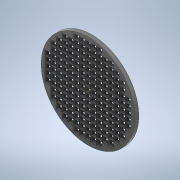
# Autodesk Inventor part: FRAME
Saved by Autodesk Inventor 2022 (Build 260153000, 153)
## iProperties
Created: 2022-02-07
Part Number: FRAME
Material: Copper
Document SubType Name: Modeling
Designer: joshw
Density: 8.94 g/cm^3
Appearance: Diamond plate - Dark Gray
Author: joshw
Autodesk Inventor part; units mm, degrees
ref_plane "YZ Plane" through (0, 0, 0) normal (1, 0, 0) x (0, 1, 0)
ref_plane "XZ Plane" through (0, 0, 0) normal (0, 1, 0) x (-1, 0, 0)
ref_plane "XY Plane" through (0, 0, 0) normal (0, 0, 1) x (1, 0, 0)
sketch "Sketch5" plane through (0, 0, 0) normal (0, 0, 1) x (1, 0, 0)
  line L0 (115, 115) -> (115, -115) construction
  line L1 (115, -115) -> (-115, -115)
  line L2 (-115, -115) -> (-115, 115)
  line L3 (97.5, -97.5) -> (97.5, -111.5)
  line L4 (97.5, -111.5) -> (111.5, -111.5)
  line L5 (111.5, -111.5) -> (111.5, -97.5)
  line L6 (111.5, -97.5) -> (97.5, -97.5)
  line L7 (115, 115) -> (-115, 115)
  line L8 (97.5, -82.5) -> (97.5, -96.5)
  line L9 (97.5, -96.5) -> (111.5, -96.5)
  line L10 (111.5, -96.5) -> (111.5, -82.5)
  line L11 (111.5, -82.5) -> (97.5, -82.5)
  line L12 (97.5, -67.5) -> (97.5, -81.5)
  line L13 (97.5, -81.5) -> (111.5, -81.5)
  line L14 (111.5, -81.5) -> (111.5, -67.5)
  line L15 (111.5, -67.5) -> (97.5, -67.5)
  line L16 (97.5, -52.5) -> (97.5, -66.5)
  line L17 (97.5, -66.5) -> (111.5, -66.5)
  line L18 (111.5, -66.5) -> (111.5, -52.5)
  line L19 (111.5, -52.5) -> (97.5, -52.5)
  line L20 (97.5, -37.5) -> (97.5, -51.5)
  line L21 (97.5, -51.5) -> (111.5, -51.5)
  line L22 (111.5, -51.5) -> (111.5, -37.5)
  line L23 (111.5, -37.5) -> (97.5, -37.5)
  line L24 (97.5, -22.5) -> (97.5, -36.5)
  line L25 (97.5, -36.5) -> (111.5, -36.5)
  line L26 (111.5, -36.5) -> (111.5, -22.5)
  line L27 (111.5, -22.5) -> (97.5, -22.5)
  line L28 (97.5, -7.5) -> (97.5, -21.5)
  line L29 (97.5, -21.5) -> (111.5, -21.5)
  line L30 (111.5, -21.5) -> (111.5, -7.5)
  line L31 (111.5, -7.5) -> (97.5, -7.5)
  line L32 (97.5, 7.5) -> (97.5, -6.5)
  line L33 (97.5, -6.5) -> (111.5, -6.5)
  line L34 (111.5, -6.5) -> (111.5, 7.5)
  line L35 (111.5, 7.5) -> (97.5, 7.5)
  line L36 (97.5, 22.5) -> (97.5, 8.5)
  line L37 (97.5, 8.5) -> (111.5, 8.5)
  line L38 (111.5, 8.5) -> (111.5, 22.5)
  line L39 (111.5, 22.5) -> (97.5, 22.5)
  line L40 (97.5, 37.5) -> (97.5, 23.5)
  line L41 (97.5, 23.5) -> (111.5, 23.5)
  line L42 (111.5, 23.5) -> (111.5, 37.5)
  line L43 (111.5, 37.5) -> (97.5, 37.5)
  line L44 (97.5, 52.5) -> (97.5, 38.5)
  line L45 (97.5, 38.5) -> (111.5, 38.5)
  line L46 (111.5, 38.5) -> (111.5, 52.5)
  line L47 (111.5, 52.5) -> (97.5, 52.5)
  line L48 (97.5, 67.5) -> (97.5, 53.5)
  line L49 (97.5, 53.5) -> (111.5, 53.5)
  line L50 (111.5, 53.5) -> (111.5, 67.5)
  line L51 (111.5, 67.5) -> (97.5, 67.5)
  line L52 (97.5, 82.5) -> (97.5, 68.5)
  line L53 (97.5, 68.5) -> (111.5, 68.5)
  line L54 (111.5, 68.5) -> (111.5, 82.5)
  line L55 (111.5, 82.5) -> (97.5, 82.5)
  line L56 (97.5, 97.5) -> (97.5, 83.5)
  line L57 (97.5, 83.5) -> (111.5, 83.5)
  line L58 (111.5, 83.5) -> (111.5, 97.5)
  line L59 (111.5, 97.5) -> (97.5, 97.5)
  line L60 (97.5, 112.5) -> (97.5, 98.5)
  line L61 (97.5, 98.5) -> (111.5, 98.5)
  line L62 (111.5, 98.5) -> (111.5, 112.5)
  line L63 (111.5, 112.5) -> (97.5, 112.5)
  line L64 (82.5, -97.5) -> (82.5, -111.5)
  line L65 (82.5, -111.5) -> (96.5, -111.5)
  line L66 (96.5, -111.5) -> (96.5, -97.5)
  line L67 (96.5, -97.5) -> (82.5, -97.5)
  line L68 (82.5, -82.5) -> (82.5, -96.5)
  line L69 (82.5, -96.5) -> (96.5, -96.5)
  line L70 (96.5, -96.5) -> (96.5, -82.5)
  line L71 (96.5, -82.5) -> (82.5, -82.5)
  line L72 (82.5, -67.5) -> (82.5, -81.5)
  line L73 (82.5, -81.5) -> (96.5, -81.5)
  line L74 (96.5, -81.5) -> (96.5, -67.5)
  line L75 (96.5, -67.5) -> (82.5, -67.5)
  line L76 (82.5, -52.5) -> (82.5, -66.5)
  line L77 (82.5, -66.5) -> (96.5, -66.5)
  line L78 (96.5, -66.5) -> (96.5, -52.5)
  line L79 (96.5, -52.5) -> (82.5, -52.5)
  line L80 (82.5, -37.5) -> (82.5, -51.5)
  line L81 (82.5, -51.5) -> (96.5, -51.5)
  line L82 (96.5, -51.5) -> (96.5, -37.5)
  line L83 (96.5, -37.5) -> (82.5, -37.5)
  line L84 (82.5, -22.5) -> (82.5, -36.5)
  line L85 (82.5, -36.5) -> (96.5, -36.5)
  line L86 (96.5, -36.5) -> (96.5, -22.5)
  line L87 (96.5, -22.5) -> (82.5, -22.5)
  line L88 (82.5, -7.5) -> (82.5, -21.5)
  line L89 (82.5, -21.5) -> (96.5, -21.5)
  line L90 (96.5, -21.5) -> (96.5, -7.5)
  line L91 (96.5, -7.5) -> (82.5, -7.5)
  line L92 (82.5, 7.5) -> (82.5, -6.5)
  line L93 (82.5, -6.5) -> (96.5, -6.5)
  line L94 (96.5, -6.5) -> (96.5, 7.5)
  line L95 (96.5, 7.5) -> (82.5, 7.5)
  line L96 (82.5, 22.5) -> (82.5, 8.5)
  line L97 (82.5, 8.5) -> (96.5, 8.5)
  line L98 (96.5, 8.5) -> (96.5, 22.5)
  line L99 (96.5, 22.5) -> (82.5, 22.5)
  line L100 (82.5, 37.5) -> (82.5, 23.5)
  line L101 (82.5, 23.5) -> (96.5, 23.5)
  line L102 (96.5, 23.5) -> (96.5, 37.5)
  line L103 (96.5, 37.5) -> (82.5, 37.5)
  line L104 (82.5, 52.5) -> (82.5, 38.5)
  line L105 (82.5, 38.5) -> (96.5, 38.5)
  line L106 (96.5, 38.5) -> (96.5, 52.5)
  line L107 (96.5, 52.5) -> (82.5, 52.5)
  line L108 (82.5, 67.5) -> (82.5, 53.5)
  line L109 (82.5, 53.5) -> (96.5, 53.5)
  line L110 (96.5, 53.5) -> (96.5, 67.5)
  line L111 (96.5, 67.5) -> (82.5, 67.5)
  line L112 (82.5, 82.5) -> (82.5, 68.5)
  line L113 (82.5, 68.5) -> (96.5, 68.5)
  line L114 (96.5, 68.5) -> (96.5, 82.5)
  line L115 (96.5, 82.5) -> (82.5, 82.5)
  line L116 (82.5, 97.5) -> (82.5, 83.5)
  line L117 (82.5, 83.5) -> (96.5, 83.5)
  line L118 (96.5, 83.5) -> (96.5, 97.5)
  line L119 (96.5, 97.5) -> (82.5, 97.5)
  line L120 (82.5, 112.5) -> (82.5, 98.5)
  line L121 (82.5, 98.5) -> (96.5, 98.5)
  line L122 (96.5, 98.5) -> (96.5, 112.5)
  line L123 (96.5, 112.5) -> (82.5, 112.5)
  line L124 (67.5, -97.5) -> (67.5, -111.5)
  line L125 (67.5, -111.5) -> (81.5, -111.5)
  line L126 (81.5, -111.5) -> (81.5, -97.5)
  line L127 (81.5, -97.5) -> (67.5, -97.5)
  line L128 (67.5, -82.5) -> (67.5, -96.5)
  line L129 (67.5, -96.5) -> (81.5, -96.5)
  line L130 (81.5, -96.5) -> (81.5, -82.5)
  line L131 (81.5, -82.5) -> (67.5, -82.5)
  line L132 (67.5, -67.5) -> (67.5, -81.5)
  line L133 (67.5, -81.5) -> (81.5, -81.5)
  line L134 (81.5, -81.5) -> (81.5, -67.5)
  line L135 (81.5, -67.5) -> (67.5, -67.5)
  line L136 (67.5, -52.5) -> (67.5, -66.5)
  line L137 (67.5, -66.5) -> (81.5, -66.5)
  line L138 (81.5, -66.5) -> (81.5, -52.5)
  line L139 (81.5, -52.5) -> (67.5, -52.5)
  line L140 (67.5, -37.5) -> (67.5, -51.5)
  line L141 (67.5, -51.5) -> (81.5, -51.5)
  line L142 (81.5, -51.5) -> (81.5, -37.5)
  line L143 (81.5, -37.5) -> (67.5, -37.5)
  line L144 (67.5, -22.5) -> (67.5, -36.5)
  line L145 (67.5, -36.5) -> (81.5, -36.5)
  line L146 (81.5, -36.5) -> (81.5, -22.5)
  line L147 (81.5, -22.5) -> (67.5, -22.5)
  line L148 (67.5, -7.5) -> (67.5, -21.5)
  line L149 (67.5, -21.5) -> (81.5, -21.5)
  line L150 (81.5, -21.5) -> (81.5, -7.5)
  line L151 (81.5, -7.5) -> (67.5, -7.5)
  line L152 (67.5, 7.5) -> (67.5, -6.5)
  line L153 (67.5, -6.5) -> (81.5, -6.5)
  line L154 (81.5, -6.5) -> (81.5, 7.5)
  line L155 (81.5, 7.5) -> (67.5, 7.5)
  line L156 (67.5, 22.5) -> (67.5, 8.5)
  line L157 (67.5, 8.5) -> (81.5, 8.5)
  line L158 (81.5, 8.5) -> (81.5, 22.5)
  line L159 (81.5, 22.5) -> (67.5, 22.5)
  line L160 (67.5, 37.5) -> (67.5, 23.5)
  line L161 (67.5, 23.5) -> (81.5, 23.5)
  line L162 (81.5, 23.5) -> (81.5, 37.5)
  line L163 (81.5, 37.5) -> (67.5, 37.5)
  line L164 (67.5, 52.5) -> (67.5, 38.5)
  line L165 (67.5, 38.5) -> (81.5, 38.5)
  line L166 (81.5, 38.5) -> (81.5, 52.5)
  line L167 (81.5, 52.5) -> (67.5, 52.5)
  line L168 (67.5, 67.5) -> (67.5, 53.5)
  line L169 (67.5, 53.5) -> (81.5, 53.5)
  line L170 (81.5, 53.5) -> (81.5, 67.5)
  line L171 (81.5, 67.5) -> (67.5, 67.5)
  line L172 (67.5, 82.5) -> (67.5, 68.5)
  line L173 (67.5, 68.5) -> (81.5, 68.5)
  line L174 (81.5, 68.5) -> (81.5, 82.5)
  line L175 (81.5, 82.5) -> (67.5, 82.5)
  line L176 (67.5, 97.5) -> (67.5, 83.5)
  line L177 (67.5, 83.5) -> (81.5, 83.5)
  line L178 (81.5, 83.5) -> (81.5, 97.5)
  line L179 (81.5, 97.5) -> (67.5, 97.5)
  line L180 (67.5, 112.5) -> (67.5, 98.5)
  line L181 (67.5, 98.5) -> (81.5, 98.5)
  line L182 (81.5, 98.5) -> (81.5, 112.5)
  line L183 (81.5, 112.5) -> (67.5, 112.5)
  line L184 (52.5, -97.5) -> (52.5, -111.5)
  line L185 (52.5, -111.5) -> (66.5, -111.5)
  line L186 (66.5, -111.5) -> (66.5, -97.5)
  line L187 (66.5, -97.5) -> (52.5, -97.5)
  line L188 (52.5, -82.5) -> (52.5, -96.5)
  line L189 (52.5, -96.5) -> (66.5, -96.5)
  line L190 (66.5, -96.5) -> (66.5, -82.5)
  line L191 (66.5, -82.5) -> (52.5, -82.5)
  line L192 (52.5, -67.5) -> (52.5, -81.5)
  line L193 (52.5, -81.5) -> (66.5, -81.5)
  line L194 (66.5, -81.5) -> (66.5, -67.5)
  line L195 (66.5, -67.5) -> (52.5, -67.5)
  line L196 (52.5, -52.5) -> (52.5, -66.5)
  line L197 (52.5, -66.5) -> (66.5, -66.5)
  line L198 (66.5, -66.5) -> (66.5, -52.5)
  line L199 (66.5, -52.5) -> (52.5, -52.5)
  line L200 (52.5, -37.5) -> (52.5, -51.5)
  line L201 (52.5, -51.5) -> (66.5, -51.5)
  line L202 (66.5, -51.5) -> (66.5, -37.5)
  line L203 (66.5, -37.5) -> (52.5, -37.5)
  line L204 (52.5, -22.5) -> (52.5, -36.5)
  line L205 (52.5, -36.5) -> (66.5, -36.5)
  line L206 (66.5, -36.5) -> (66.5, -22.5)
  line L207 (66.5, -22.5) -> (52.5, -22.5)
  line L208 (52.5, -7.5) -> (52.5, -21.5)
  line L209 (52.5, -21.5) -> (66.5, -21.5)
  line L210 (66.5, -21.5) -> (66.5, -7.5)
  line L211 (66.5, -7.5) -> (52.5, -7.5)
  line L212 (52.5, 7.5) -> (52.5, -6.5)
  line L213 (52.5, -6.5) -> (66.5, -6.5)
  line L214 (66.5, -6.5) -> (66.5, 7.5)
  line L215 (66.5, 7.5) -> (52.5, 7.5)
  line L216 (52.5, 22.5) -> (52.5, 8.5)
  line L217 (52.5, 8.5) -> (66.5, 8.5)
  line L218 (66.5, 8.5) -> (66.5, 22.5)
  line L219 (66.5, 22.5) -> (52.5, 22.5)
  line L220 (52.5, 37.5) -> (52.5, 23.5)
  line L221 (52.5, 23.5) -> (66.5, 23.5)
  line L222 (66.5, 23.5) -> (66.5, 37.5)
  line L223 (66.5, 37.5) -> (52.5, 37.5)
  line L224 (52.5, 52.5) -> (52.5, 38.5)
  line L225 (52.5, 38.5) -> (66.5, 38.5)
  line L226 (66.5, 38.5) -> (66.5, 52.5)
  line L227 (66.5, 52.5) -> (52.5, 52.5)
  line L228 (52.5, 67.5) -> (52.5, 53.5)
  line L229 (52.5, 53.5) -> (66.5, 53.5)
  line L230 (66.5, 53.5) -> (66.5, 67.5)
  line L231 (66.5, 67.5) -> (52.5, 67.5)
  line L232 (52.5, 82.5) -> (52.5, 68.5)
  line L233 (52.5, 68.5) -> (66.5, 68.5)
  line L234 (66.5, 68.5) -> (66.5, 82.5)
  line L235 (66.5, 82.5) -> (52.5, 82.5)
  line L236 (52.5, 97.5) -> (52.5, 83.5)
  line L237 (52.5, 83.5) -> (66.5, 83.5)
  line L238 (66.5, 83.5) -> (66.5, 97.5)
  line L239 (66.5, 97.5) -> (52.5, 97.5)
  line L240 (52.5, 112.5) -> (52.5, 98.5)
  line L241 (52.5, 98.5) -> (66.5, 98.5)
  line L242 (66.5, 98.5) -> (66.5, 112.5)
  line L243 (66.5, 112.5) -> (52.5, 112.5)
  line L244 (37.5, -97.5) -> (37.5, -111.5)
  line L245 (37.5, -111.5) -> (51.5, -111.5)
  line L246 (51.5, -111.5) -> (51.5, -97.5)
  line L247 (51.5, -97.5) -> (37.5, -97.5)
  line L248 (37.5, -82.5) -> (37.5, -96.5)
  line L249 (37.5, -96.5) -> (51.5, -96.5)
  line L250 (51.5, -96.5) -> (51.5, -82.5)
  line L251 (51.5, -82.5) -> (37.5, -82.5)
  line L252 (37.5, -67.5) -> (37.5, -81.5)
  line L253 (37.5, -81.5) -> (51.5, -81.5)
  line L254 (51.5, -81.5) -> (51.5, -67.5)
  line L255 (51.5, -67.5) -> (37.5, -67.5)
  line L256 (37.5, -52.5) -> (37.5, -66.5)
  line L257 (37.5, -66.5) -> (51.5, -66.5)
  line L258 (51.5, -66.5) -> (51.5, -52.5)
  line L259 (51.5, -52.5) -> (37.5, -52.5)
  line L260 (37.5, -37.5) -> (37.5, -51.5)
  line L261 (37.5, -51.5) -> (51.5, -51.5)
  line L262 (51.5, -51.5) -> (51.5, -37.5)
  line L263 (51.5, -37.5) -> (37.5, -37.5)
  line L264 (37.5, -22.5) -> (37.5, -36.5)
  line L265 (37.5, -36.5) -> (51.5, -36.5)
  line L266 (51.5, -36.5) -> (51.5, -22.5)
  line L267 (51.5, -22.5) -> (37.5, -22.5)
  line L268 (37.5, -7.5) -> (37.5, -21.5)
  line L269 (37.5, -21.5) -> (51.5, -21.5)
  line L270 (51.5, -21.5) -> (51.5, -7.5)
  line L271 (51.5, -7.5) -> (37.5, -7.5)
  line L272 (37.5, 7.5) -> (37.5, -6.5)
  line L273 (37.5, -6.5) -> (51.5, -6.5)
  line L274 (51.5, -6.5) -> (51.5, 7.5)
  line L275 (51.5, 7.5) -> (37.5, 7.5)
  line L276 (37.5, 22.5) -> (37.5, 8.5)
  line L277 (37.5, 8.5) -> (51.5, 8.5)
  line L278 (51.5, 8.5) -> (51.5, 22.5)
  line L279 (51.5, 22.5) -> (37.5, 22.5)
  line L280 (37.5, 37.5) -> (37.5, 23.5)
  line L281 (37.5, 23.5) -> (51.5, 23.5)
  line L282 (51.5, 23.5) -> (51.5, 37.5)
  line L283 (51.5, 37.5) -> (37.5, 37.5)
  line L284 (37.5, 52.5) -> (37.5, 38.5)
  line L285 (37.5, 38.5) -> (51.5, 38.5)
  line L286 (51.5, 38.5) -> (51.5, 52.5)
  line L287 (51.5, 52.5) -> (37.5, 52.5)
  line L288 (37.5, 67.5) -> (37.5, 53.5)
  line L289 (37.5, 53.5) -> (51.5, 53.5)
  line L290 (51.5, 53.5) -> (51.5, 67.5)
  line L291 (51.5, 67.5) -> (37.5, 67.5)
  line L292 (37.5, 82.5) -> (37.5, 68.5)
  line L293 (37.5, 68.5) -> (51.5, 68.5)
  line L294 (51.5, 68.5) -> (51.5, 82.5)
  line L295 (51.5, 82.5) -> (37.5, 82.5)
  line L296 (37.5, 97.5) -> (37.5, 83.5)
  line L297 (37.5, 83.5) -> (51.5, 83.5)
  line L298 (51.5, 83.5) -> (51.5, 97.5)
  line L299 (51.5, 97.5) -> (37.5, 97.5)
  line L300 (37.5, 112.5) -> (37.5, 98.5)
  line L301 (37.5, 98.5) -> (51.5, 98.5)
  line L302 (51.5, 98.5) -> (51.5, 112.5)
  line L303 (51.5, 112.5) -> (37.5, 112.5)
  line L304 (22.5, -97.5) -> (22.5, -111.5)
  line L305 (22.5, -111.5) -> (36.5, -111.5)
  line L306 (36.5, -111.5) -> (36.5, -97.5)
  line L307 (36.5, -97.5) -> (22.5, -97.5)
  line L308 (22.5, -82.5) -> (22.5, -96.5)
  line L309 (22.5, -96.5) -> (36.5, -96.5)
  line L310 (36.5, -96.5) -> (36.5, -82.5)
  line L311 (36.5, -82.5) -> (22.5, -82.5)
  line L312 (22.5, -67.5) -> (22.5, -81.5)
  line L313 (22.5, -81.5) -> (36.5, -81.5)
  line L314 (36.5, -81.5) -> (36.5, -67.5)
  line L315 (36.5, -67.5) -> (22.5, -67.5)
  line L316 (22.5, -52.5) -> (22.5, -66.5)
  line L317 (22.5, -66.5) -> (36.5, -66.5)
  line L318 (36.5, -66.5) -> (36.5, -52.5)
  line L319 (36.5, -52.5) -> (22.5, -52.5)
  line L320 (22.5, -37.5) -> (22.5, -51.5)
  line L321 (22.5, -51.5) -> (36.5, -51.5)
  line L322 (36.5, -51.5) -> (36.5, -37.5)
  line L323 (36.5, -37.5) -> (22.5, -37.5)
  line L324 (22.5, -22.5) -> (22.5, -36.5)
  line L325 (22.5, -36.5) -> (36.5, -36.5)
  line L326 (36.5, -36.5) -> (36.5, -22.5)
  line L327 (36.5, -22.5) -> (22.5, -22.5)
  line L328 (22.5, -7.5) -> (22.5, -21.5)
  line L329 (22.5, -21.5) -> (36.5, -21.5)
  line L330 (36.5, -21.5) -> (36.5, -7.5)
  line L331 (36.5, -7.5) -> (22.5, -7.5)
  line L332 (22.5, 7.5) -> (22.5, -6.5)
  line L333 (22.5, -6.5) -> (36.5, -6.5)
  line L334 (36.5, -6.5) -> (36.5, 7.5)
  line L335 (36.5, 7.5) -> (22.5, 7.5)
  line L336 (22.5, 22.5) -> (22.5, 8.5)
  line L337 (22.5, 8.5) -> (36.5, 8.5)
  line L338 (36.5, 8.5) -> (36.5, 22.5)
  line L339 (36.5, 22.5) -> (22.5, 22.5)
  line L340 (22.5, 37.5) -> (22.5, 23.5)
  line L341 (22.5, 23.5) -> (36.5, 23.5)
  line L342 (36.5, 23.5) -> (36.5, 37.5)
  line L343 (36.5, 37.5) -> (22.5, 37.5)
  line L344 (22.5, 52.5) -> (22.5, 38.5)
  line L345 (22.5, 38.5) -> (36.5, 38.5)
  line L346 (36.5, 38.5) -> (36.5, 52.5)
  line L347 (36.5, 52.5) -> (22.5, 52.5)
  line L348 (22.5, 67.5) -> (22.5, 53.5)
  line L349 (22.5, 53.5) -> (36.5, 53.5)
  line L350 (36.5, 53.5) -> (36.5, 67.5)
  line L351 (36.5, 67.5) -> (22.5, 67.5)
  line L352 (22.5, 82.5) -> (22.5, 68.5)
  line L353 (22.5, 68.5) -> (36.5, 68.5)
  line L354 (36.5, 68.5) -> (36.5, 82.5)
  line L355 (36.5, 82.5) -> (22.5, 82.5)
  line L356 (22.5, 97.5) -> (22.5, 83.5)
  line L357 (22.5, 83.5) -> (36.5, 83.5)
  line L358 (36.5, 83.5) -> (36.5, 97.5)
  line L359 (36.5, 97.5) -> (22.5, 97.5)
  line L360 (22.5, 112.5) -> (22.5, 98.5)
  line L361 (22.5, 98.5) -> (36.5, 98.5)
  line L362 (36.5, 98.5) -> (36.5, 112.5)
  line L363 (36.5, 112.5) -> (22.5, 112.5)
  line L364 (7.5, -97.5) -> (7.5, -111.5)
  line L365 (7.5, -111.5) -> (21.5, -111.5)
  line L366 (21.5, -111.5) -> (21.5, -97.5)
  line L367 (21.5, -97.5) -> (7.5, -97.5)
  line L368 (7.5, -82.5) -> (7.5, -96.5)
  line L369 (7.5, -96.5) -> (21.5, -96.5)
  line L370 (21.5, -96.5) -> (21.5, -82.5)
  line L371 (21.5, -82.5) -> (7.5, -82.5)
  line L372 (7.5, -67.5) -> (7.5, -81.5)
  line L373 (7.5, -81.5) -> (21.5, -81.5)
  line L374 (21.5, -81.5) -> (21.5, -67.5)
  line L375 (21.5, -67.5) -> (7.5, -67.5)
  line L376 (7.5, -52.5) -> (7.5, -66.5)
  line L377 (7.5, -66.5) -> (21.5, -66.5)
  line L378 (21.5, -66.5) -> (21.5, -52.5)
  line L379 (21.5, -52.5) -> (7.5, -52.5)
  line L380 (7.5, -37.5) -> (7.5, -51.5)
  line L381 (7.5, -51.5) -> (21.5, -51.5)
  line L382 (21.5, -51.5) -> (21.5, -37.5)
  line L383 (21.5, -37.5) -> (7.5, -37.5)
  line L384 (7.5, -22.5) -> (7.5, -36.5)
  line L385 (7.5, -36.5) -> (21.5, -36.5)
  line L386 (21.5, -36.5) -> (21.5, -22.5)
  line L387 (21.5, -22.5) -> (7.5, -22.5)
  line L388 (7.5, -7.5) -> (7.5, -21.5)
  line L389 (7.5, -21.5) -> (21.5, -21.5)
  line L390 (21.5, -21.5) -> (21.5, -7.5)
  line L391 (21.5, -7.5) -> (7.5, -7.5)
  line L392 (7.5, 7.5) -> (7.5, -6.5)
  line L393 (7.5, -6.5) -> (21.5, -6.5)
  line L394 (21.5, -6.5) -> (21.5, 7.5)
  line L395 (21.5, 7.5) -> (7.5, 7.5)
  line L396 (7.5, 22.5) -> (7.5, 8.5)
  line L397 (7.5, 8.5) -> (21.5, 8.5)
  line L398 (21.5, 8.5) -> (21.5, 22.5)
  line L399 (21.5, 22.5) -> (7.5, 22.5)
  line L400 (7.5, 37.5) -> (7.5, 23.5)
  line L401 (7.5, 23.5) -> (21.5, 23.5)
  line L402 (21.5, 23.5) -> (21.5, 37.5)
  line L403 (21.5, 37.5) -> (7.5, 37.5)
  line L404 (7.5, 52.5) -> (7.5, 38.5)
  line L405 (7.5, 38.5) -> (21.5, 38.5)
  line L406 (21.5, 38.5) -> (21.5, 52.5)
  line L407 (21.5, 52.5) -> (7.5, 52.5)
  line L408 (7.5, 67.5) -> (7.5, 53.5)
  line L409 (7.5, 53.5) -> (21.5, 53.5)
  line L410 (21.5, 53.5) -> (21.5, 67.5)
  line L411 (21.5, 67.5) -> (7.5, 67.5)
  line L412 (7.5, 82.5) -> (7.5, 68.5)
  line L413 (7.5, 68.5) -> (21.5, 68.5)
  line L414 (21.5, 68.5) -> (21.5, 82.5)
  line L415 (21.5, 82.5) -> (7.5, 82.5)
  line L416 (7.5, 97.5) -> (7.5, 83.5)
  line L417 (7.5, 83.5) -> (21.5, 83.5)
  line L418 (21.5, 83.5) -> (21.5, 97.5)
  line L419 (21.5, 97.5) -> (7.5, 97.5)
  line L420 (7.5, 112.5) -> (7.5, 98.5)
  line L421 (7.5, 98.5) -> (21.5, 98.5)
  line L422 (21.5, 98.5) -> (21.5, 112.5)
  line L423 (21.5, 112.5) -> (7.5, 112.5)
  line L424 (-7.5, -97.5) -> (-7.5, -111.5)
  line L425 (-7.5, -111.5) -> (6.5, -111.5)
  line L426 (6.5, -111.5) -> (6.5, -97.5)
  line L427 (6.5, -97.5) -> (-7.5, -97.5)
  line L428 (-7.5, -82.5) -> (-7.5, -96.5)
  line L429 (-7.5, -96.5) -> (6.5, -96.5)
  line L430 (6.5, -96.5) -> (6.5, -82.5)
  line L431 (6.5, -82.5) -> (-7.5, -82.5)
  line L432 (-7.5, -67.5) -> (-7.5, -81.5)
  line L433 (-7.5, -81.5) -> (6.5, -81.5)
  line L434 (6.5, -81.5) -> (6.5, -67.5)
  line L435 (6.5, -67.5) -> (-7.5, -67.5)
  line L436 (-7.5, -52.5) -> (-7.5, -66.5)
  line L437 (-7.5, -66.5) -> (6.5, -66.5)
  line L438 (6.5, -66.5) -> (6.5, -52.5)
  line L439 (6.5, -52.5) -> (-7.5, -52.5)
  line L440 (-7.5, -37.5) -> (-7.5, -51.5)
  line L441 (-7.5, -51.5) -> (6.5, -51.5)
  line L442 (6.5, -51.5) -> (6.5, -37.5)
  line L443 (6.5, -37.5) -> (-7.5, -37.5)
  line L444 (-7.5, -22.5) -> (-7.5, -36.5)
  line L445 (-7.5, -36.5) -> (6.5, -36.5)
  line L446 (6.5, -36.5) -> (6.5, -22.5)
  line L447 (6.5, -22.5) -> (-7.5, -22.5)
  line L448 (-7.5, -7.5) -> (-7.5, -21.5)
  line L449 (-7.5, -21.5) -> (6.5, -21.5)
  line L450 (6.5, -21.5) -> (6.5, -7.5)
  line L451 (6.5, -7.5) -> (-7.5, -7.5)
  line L452 (-7.5, 7.5) -> (-7.5, -6.5)
  line L453 (-7.5, -6.5) -> (6.5, -6.5)
  line L454 (6.5, -6.5) -> (6.5, 7.5)
  line L455 (6.5, 7.5) -> (-7.5, 7.5)
  line L456 (-7.5, 22.5) -> (-7.5, 8.5)
  line L457 (-7.5, 8.5) -> (6.5, 8.5)
  line L458 (6.5, 8.5) -> (6.5, 22.5)
  line L459 (6.5, 22.5) -> (-7.5, 22.5)
  line L460 (-7.5, 37.5) -> (-7.5, 23.5)
  line L461 (-7.5, 23.5) -> (6.5, 23.5)
  line L462 (6.5, 23.5) -> (6.5, 37.5)
  line L463 (6.5, 37.5) -> (-7.5, 37.5)
  line L464 (-7.5, 52.5) -> (-7.5, 38.5)
  line L465 (-7.5, 38.5) -> (6.5, 38.5)
  line L466 (6.5, 38.5) -> (6.5, 52.5)
  line L467 (6.5, 52.5) -> (-7.5, 52.5)
  line L468 (-7.5, 67.5) -> (-7.5, 53.5)
  line L469 (-7.5, 53.5) -> (6.5, 53.5)
  line L470 (6.5, 53.5) -> (6.5, 67.5)
  line L471 (6.5, 67.5) -> (-7.5, 67.5)
  line L472 (-7.5, 82.5) -> (-7.5, 68.5)
  line L473 (-7.5, 68.5) -> (6.5, 68.5)
  line L474 (6.5, 68.5) -> (6.5, 82.5)
  line L475 (6.5, 82.5) -> (-7.5, 82.5)
  line L476 (-7.5, 97.5) -> (-7.5, 83.5)
  line L477 (-7.5, 83.5) -> (6.5, 83.5)
  line L478 (6.5, 83.5) -> (6.5, 97.5)
  line L479 (6.5, 97.5) -> (-7.5, 97.5)
  line L480 (-7.5, 112.5) -> (-7.5, 98.5)
  line L481 (-7.5, 98.5) -> (6.5, 98.5)
  line L482 (6.5, 98.5) -> (6.5, 112.5)
  line L483 (6.5, 112.5) -> (-7.5, 112.5)
  line L484 (-22.5, -97.5) -> (-22.5, -111.5)
  line L485 (-22.5, -111.5) -> (-8.5, -111.5)
  line L486 (-8.5, -111.5) -> (-8.5, -97.5)
  line L487 (-8.5, -97.5) -> (-22.5, -97.5)
  line L488 (-22.5, -82.5) -> (-22.5, -96.5)
  line L489 (-22.5, -96.5) -> (-8.5, -96.5)
  line L490 (-8.5, -96.5) -> (-8.5, -82.5)
  line L491 (-8.5, -82.5) -> (-22.5, -82.5)
  line L492 (-22.5, -67.5) -> (-22.5, -81.5)
  line L493 (-22.5, -81.5) -> (-8.5, -81.5)
  line L494 (-8.5, -81.5) -> (-8.5, -67.5)
  line L495 (-8.5, -67.5) -> (-22.5, -67.5)
  line L496 (-22.5, -52.5) -> (-22.5, -66.5)
  line L497 (-22.5, -66.5) -> (-8.5, -66.5)
  line L498 (-8.5, -66.5) -> (-8.5, -52.5)
  line L499 (-8.5, -52.5) -> (-22.5, -52.5)
  line L500 (-22.5, -37.5) -> (-22.5, -51.5)
  line L501 (-22.5, -51.5) -> (-8.5, -51.5)
  line L502 (-8.5, -51.5) -> (-8.5, -37.5)
  line L503 (-8.5, -37.5) -> (-22.5, -37.5)
  line L504 (-22.5, -22.5) -> (-22.5, -36.5)
  line L505 (-22.5, -36.5) -> (-8.5, -36.5)
  line L506 (-8.5, -36.5) -> (-8.5, -22.5)
  line L507 (-8.5, -22.5) -> (-22.5, -22.5)
  line L508 (-22.5, -7.5) -> (-22.5, -21.5)
  line L509 (-22.5, -21.5) -> (-8.5, -21.5)
  line L510 (-8.5, -21.5) -> (-8.5, -7.5)
  line L511 (-8.5, -7.5) -> (-22.5, -7.5)
  line L512 (-22.5, 7.5) -> (-22.5, -6.5)
  line L513 (-22.5, -6.5) -> (-8.5, -6.5)
  line L514 (-8.5, -6.5) -> (-8.5, 7.5)
  line L515 (-8.5, 7.5) -> (-22.5, 7.5)
  line L516 (-22.5, 22.5) -> (-22.5, 8.5)
  line L517 (-22.5, 8.5) -> (-8.5, 8.5)
  line L518 (-8.5, 8.5) -> (-8.5, 22.5)
  line L519 (-8.5, 22.5) -> (-22.5, 22.5)
  line L520 (-22.5, 37.5) -> (-22.5, 23.5)
  line L521 (-22.5, 23.5) -> (-8.5, 23.5)
  line L522 (-8.5, 23.5) -> (-8.5, 37.5)
  line L523 (-8.5, 37.5) -> (-22.5, 37.5)
  line L524 (-22.5, 52.5) -> (-22.5, 38.5)
  line L525 (-22.5, 38.5) -> (-8.5, 38.5)
  line L526 (-8.5, 38.5) -> (-8.5, 52.5)
  line L527 (-8.5, 52.5) -> (-22.5, 52.5)
  line L528 (-22.5, 67.5) -> (-22.5, 53.5)
  line L529 (-22.5, 53.5) -> (-8.5, 53.5)
  line L530 (-8.5, 53.5) -> (-8.5, 67.5)
  line L531 (-8.5, 67.5) -> (-22.5, 67.5)
  line L532 (-22.5, 82.5) -> (-22.5, 68.5)
  line L533 (-22.5, 68.5) -> (-8.5, 68.5)
  line L534 (-8.5, 68.5) -> (-8.5, 82.5)
  line L535 (-8.5, 82.5) -> (-22.5, 82.5)
  line L536 (-22.5, 97.5) -> (-22.5, 83.5)
  line L537 (-22.5, 83.5) -> (-8.5, 83.5)
  line L538 (-8.5, 83.5) -> (-8.5, 97.5)
  line L539 (-8.5, 97.5) -> (-22.5, 97.5)
  line L540 (-22.5, 112.5) -> (-22.5, 98.5)
  line L541 (-22.5, 98.5) -> (-8.5, 98.5)
  line L542 (-8.5, 98.5) -> (-8.5, 112.5)
  line L543 (-8.5, 112.5) -> (-22.5, 112.5)
  line L544 (-37.5, -97.5) -> (-37.5, -111.5)
  line L545 (-37.5, -111.5) -> (-23.5, -111.5)
  line L546 (-23.5, -111.5) -> (-23.5, -97.5)
  line L547 (-23.5, -97.5) -> (-37.5, -97.5)
  line L548 (-37.5, -82.5) -> (-37.5, -96.5)
  line L549 (-37.5, -96.5) -> (-23.5, -96.5)
  line L550 (-23.5, -96.5) -> (-23.5, -82.5)
  line L551 (-23.5, -82.5) -> (-37.5, -82.5)
  line L552 (-37.5, -67.5) -> (-37.5, -81.5)
  line L553 (-37.5, -81.5) -> (-23.5, -81.5)
  line L554 (-23.5, -81.5) -> (-23.5, -67.5)
  line L555 (-23.5, -67.5) -> (-37.5, -67.5)
  line L556 (-37.5, -52.5) -> (-37.5, -66.5)
  line L557 (-37.5, -66.5) -> (-23.5, -66.5)
  line L558 (-23.5, -66.5) -> (-23.5, -52.5)
  line L559 (-23.5, -52.5) -> (-37.5, -52.5)
  line L560 (-37.5, -37.5) -> (-37.5, -51.5)
  line L561 (-37.5, -51.5) -> (-23.5, -51.5)
  line L562 (-23.5, -51.5) -> (-23.5, -37.5)
  line L563 (-23.5, -37.5) -> (-37.5, -37.5)
  line L564 (-37.5, -22.5) -> (-37.5, -36.5)
  line L565 (-37.5, -36.5) -> (-23.5, -36.5)
  line L566 (-23.5, -36.5) -> (-23.5, -22.5)
  line L567 (-23.5, -22.5) -> (-37.5, -22.5)
  line L568 (-37.5, -7.5) -> (-37.5, -21.5)
  line L569 (-37.5, -21.5) -> (-23.5, -21.5)
  line L570 (-23.5, -21.5) -> (-23.5, -7.5)
  line L571 (-23.5, -7.5) -> (-37.5, -7.5)
  line L572 (-37.5, 7.5) -> (-37.5, -6.5)
  line L573 (-37.5, -6.5) -> (-23.5, -6.5)
  line L574 (-23.5, -6.5) -> (-23.5, 7.5)
  line L575 (-23.5, 7.5) -> (-37.5, 7.5)
  line L576 (-37.5, 22.5) -> (-37.5, 8.5)
  line L577 (-37.5, 8.5) -> (-23.5, 8.5)
  line L578 (-23.5, 8.5) -> (-23.5, 22.5)
  line L579 (-23.5, 22.5) -> (-37.5, 22.5)
  line L580 (-37.5, 37.5) -> (-37.5, 23.5)
  line L581 (-37.5, 23.5) -> (-23.5, 23.5)
  line L582 (-23.5, 23.5) -> (-23.5, 37.5)
  line L583 (-23.5, 37.5) -> (-37.5, 37.5)
  line L584 (-37.5, 52.5) -> (-37.5, 38.5)
  line L585 (-37.5, 38.5) -> (-23.5, 38.5)
  line L586 (-23.5, 38.5) -> (-23.5, 52.5)
  line L587 (-23.5, 52.5) -> (-37.5, 52.5)
  line L588 (-37.5, 67.5) -> (-37.5, 53.5)
  line L589 (-37.5, 53.5) -> (-23.5, 53.5)
  line L590 (-23.5, 53.5) -> (-23.5, 67.5)
  line L591 (-23.5, 67.5) -> (-37.5, 67.5)
  line L592 (-37.5, 82.5) -> (-37.5, 68.5)
  line L593 (-37.5, 68.5) -> (-23.5, 68.5)
  line L594 (-23.5, 68.5) -> (-23.5, 82.5)
  line L595 (-23.5, 82.5) -> (-37.5, 82.5)
  line L596 (-37.5, 97.5) -> (-37.5, 83.5)
  line L597 (-37.5, 83.5) -> (-23.5, 83.5)
  line L598 (-23.5, 83.5) -> (-23.5, 97.5)
  line L599 (-23.5, 97.5) -> (-37.5, 97.5)
  line L600 (-37.5, 112.5) -> (-37.5, 98.5)
  line L601 (-37.5, 98.5) -> (-23.5, 98.5)
  line L602 (-23.5, 98.5) -> (-23.5, 112.5)
  line L603 (-23.5, 112.5) -> (-37.5, 112.5)
  line L604 (-52.5, -97.5) -> (-52.5, -111.5)
  line L605 (-52.5, -111.5) -> (-38.5, -111.5)
  line L606 (-38.5, -111.5) -> (-38.5, -97.5)
  line L607 (-38.5, -97.5) -> (-52.5, -97.5)
  line L608 (-52.5, -82.5) -> (-52.5, -96.5)
  line L609 (-52.5, -96.5) -> (-38.5, -96.5)
  line L610 (-38.5, -96.5) -> (-38.5, -82.5)
  line L611 (-38.5, -82.5) -> (-52.5, -82.5)
  line L612 (-52.5, -67.5) -> (-52.5, -81.5)
  line L613 (-52.5, -81.5) -> (-38.5, -81.5)
  line L614 (-38.5, -81.5) -> (-38.5, -67.5)
  line L615 (-38.5, -67.5) -> (-52.5, -67.5)
  line L616 (-52.5, -52.5) -> (-52.5, -66.5)
  line L617 (-52.5, -66.5) -> (-38.5, -66.5)
  line L618 (-38.5, -66.5) -> (-38.5, -52.5)
  line L619 (-38.5, -52.5) -> (-52.5, -52.5)
  line L620 (-52.5, -37.5) -> (-52.5, -51.5)
  line L621 (-52.5, -51.5) -> (-38.5, -51.5)
  line L622 (-38.5, -51.5) -> (-38.5, -37.5)
  line L623 (-38.5, -37.5) -> (-52.5, -37.5)
  line L624 (-52.5, -22.5) -> (-52.5, -36.5)
  line L625 (-52.5, -36.5) -> (-38.5, -36.5)
  line L626 (-38.5, -36.5) -> (-38.5, -22.5)
  line L627 (-38.5, -22.5) -> (-52.5, -22.5)
  line L628 (-52.5, -7.5) -> (-52.5, -21.5)
  line L629 (-52.5, -21.5) -> (-38.5, -21.5)
  line L630 (-38.5, -21.5) -> (-38.5, -7.5)
  line L631 (-38.5, -7.5) -> (-52.5, -7.5)
  line L632 (-52.5, 7.5) -> (-52.5, -6.5)
  line L633 (-52.5, -6.5) -> (-38.5, -6.5)
  line L634 (-38.5, -6.5) -> (-38.5, 7.5)
  line L635 (-38.5, 7.5) -> (-52.5, 7.5)
  line L636 (-52.5, 22.5) -> (-52.5, 8.5)
  line L637 (-52.5, 8.5) -> (-38.5, 8.5)
  line L638 (-38.5, 8.5) -> (-38.5, 22.5)
  line L639 (-38.5, 22.5) -> (-52.5, 22.5)
  line L640 (-52.5, 37.5) -> (-52.5, 23.5)
  line L641 (-52.5, 23.5) -> (-38.5, 23.5)
  line L642 (-38.5, 23.5) -> (-38.5, 37.5)
  line L643 (-38.5, 37.5) -> (-52.5, 37.5)
  line L644 (-52.5, 52.5) -> (-52.5, 38.5)
  line L645 (-52.5, 38.5) -> (-38.5, 38.5)
  line L646 (-38.5, 38.5) -> (-38.5, 52.5)
  line L647 (-38.5, 52.5) -> (-52.5, 52.5)
  line L648 (-52.5, 67.5) -> (-52.5, 53.5)
  line L649 (-52.5, 53.5) -> (-38.5, 53.5)
  line L650 (-38.5, 53.5) -> (-38.5, 67.5)
  line L651 (-38.5, 67.5) -> (-52.5, 67.5)
  line L652 (-52.5, 82.5) -> (-52.5, 68.5)
  line L653 (-52.5, 68.5) -> (-38.5, 68.5)
  line L654 (-38.5, 68.5) -> (-38.5, 82.5)
  line L655 (-38.5, 82.5) -> (-52.5, 82.5)
  line L656 (-52.5, 97.5) -> (-52.5, 83.5)
  line L657 (-52.5, 83.5) -> (-38.5, 83.5)
  line L658 (-38.5, 83.5) -> (-38.5, 97.5)
  line L659 (-38.5, 97.5) -> (-52.5, 97.5)
  line L660 (-52.5, 112.5) -> (-52.5, 98.5)
  line L661 (-52.5, 98.5) -> (-38.5, 98.5)
  line L662 (-38.5, 98.5) -> (-38.5, 112.5)
  line L663 (-38.5, 112.5) -> (-52.5, 112.5)
  line L664 (-67.5, -97.5) -> (-67.5, -111.5)
  line L665 (-67.5, -111.5) -> (-53.5, -111.5)
  line L666 (-53.5, -111.5) -> (-53.5, -97.5)
  line L667 (-53.5, -97.5) -> (-67.5, -97.5)
  line L668 (-67.5, -82.5) -> (-67.5, -96.5)
  line L669 (-67.5, -96.5) -> (-53.5, -96.5)
  line L670 (-53.5, -96.5) -> (-53.5, -82.5)
  line L671 (-53.5, -82.5) -> (-67.5, -82.5)
  line L672 (-67.5, -67.5) -> (-67.5, -81.5)
  line L673 (-67.5, -81.5) -> (-53.5, -81.5)
  line L674 (-53.5, -81.5) -> (-53.5, -67.5)
  line L675 (-53.5, -67.5) -> (-67.5, -67.5)
  line L676 (-67.5, -52.5) -> (-67.5, -66.5)
  line L677 (-67.5, -66.5) -> (-53.5, -66.5)
  line L678 (-53.5, -66.5) -> (-53.5, -52.5)
  line L679 (-53.5, -52.5) -> (-67.5, -52.5)
  line L680 (-67.5, -37.5) -> (-67.5, -51.5)
  line L681 (-67.5, -51.5) -> (-53.5, -51.5)
  line L682 (-53.5, -51.5) -> (-53.5, -37.5)
  line L683 (-53.5, -37.5) -> (-67.5, -37.5)
  line L684 (-67.5, -22.5) -> (-67.5, -36.5)
  line L685 (-67.5, -36.5) -> (-53.5, -36.5)
  line L686 (-53.5, -36.5) -> (-53.5, -22.5)
  line L687 (-53.5, -22.5) -> (-67.5, -22.5)
  line L688 (-67.5, -7.5) -> (-67.5, -21.5)
  line L689 (-67.5, -21.5) -> (-53.5, -21.5)
  line L690 (-53.5, -21.5) -> (-53.5, -7.5)
  line L691 (-53.5, -7.5) -> (-67.5, -7.5)
  line L692 (-67.5, 7.5) -> (-67.5, -6.5)
  line L693 (-67.5, -6.5) -> (-53.5, -6.5)
  line L694 (-53.5, -6.5) -> (-53.5, 7.5)
  line L695 (-53.5, 7.5) -> (-67.5, 7.5)
  line L696 (-67.5, 22.5) -> (-67.5, 8.5)
  line L697 (-67.5, 8.5) -> (-53.5, 8.5)
  line L698 (-53.5, 8.5) -> (-53.5, 22.5)
  line L699 (-53.5, 22.5) -> (-67.5, 22.5)
  line L700 (-67.5, 37.5) -> (-67.5, 23.5)
  line L701 (-67.5, 23.5) -> (-53.5, 23.5)
  line L702 (-53.5, 23.5) -> (-53.5, 37.5)
  line L703 (-53.5, 37.5) -> (-67.5, 37.5)
  line L704 (-67.5, 52.5) -> (-67.5, 38.5)
  line L705 (-67.5, 38.5) -> (-53.5, 38.5)
  line L706 (-53.5, 38.5) -> (-53.5, 52.5)
  line L707 (-53.5, 52.5) -> (-67.5, 52.5)
  line L708 (-67.5, 67.5) -> (-67.5, 53.5)
  line L709 (-67.5, 53.5) -> (-53.5, 53.5)
  line L710 (-53.5, 53.5) -> (-53.5, 67.5)
  line L711 (-53.5, 67.5) -> (-67.5, 67.5)
  line L712 (-67.5, 82.5) -> (-67.5, 68.5)
  line L713 (-67.5, 68.5) -> (-53.5, 68.5)
  line L714 (-53.5, 68.5) -> (-53.5, 82.5)
  line L715 (-53.5, 82.5) -> (-67.5, 82.5)
  line L716 (-67.5, 97.5) -> (-67.5, 83.5)
  line L717 (-67.5, 83.5) -> (-53.5, 83.5)
  line L718 (-53.5, 83.5) -> (-53.5, 97.5)
  line L719 (-53.5, 97.5) -> (-67.5, 97.5)
  line L720 (-67.5, 112.5) -> (-67.5, 98.5)
  line L721 (-67.5, 98.5) -> (-53.5, 98.5)
  line L722 (-53.5, 98.5) -> (-53.5, 112.5)
  line L723 (-53.5, 112.5) -> (-67.5, 112.5)
  line L724 (-82.5, -97.5) -> (-82.5, -111.5)
  line L725 (-82.5, -111.5) -> (-68.5, -111.5)
  line L726 (-68.5, -111.5) -> (-68.5, -97.5)
  line L727 (-68.5, -97.5) -> (-82.5, -97.5)
  line L728 (-82.5, -82.5) -> (-82.5, -96.5)
  line L729 (-82.5, -96.5) -> (-68.5, -96.5)
  line L730 (-68.5, -96.5) -> (-68.5, -82.5)
  line L731 (-68.5, -82.5) -> (-82.5, -82.5)
  line L732 (-82.5, -67.5) -> (-82.5, -81.5)
  line L733 (-82.5, -81.5) -> (-68.5, -81.5)
  line L734 (-68.5, -81.5) -> (-68.5, -67.5)
  line L735 (-68.5, -67.5) -> (-82.5, -67.5)
  line L736 (-82.5, -52.5) -> (-82.5, -66.5)
  line L737 (-82.5, -66.5) -> (-68.5, -66.5)
  line L738 (-68.5, -66.5) -> (-68.5, -52.5)
  line L739 (-68.5, -52.5) -> (-82.5, -52.5)
  line L740 (-82.5, -37.5) -> (-82.5, -51.5)
  line L741 (-82.5, -51.5) -> (-68.5, -51.5)
  line L742 (-68.5, -51.5) -> (-68.5, -37.5)
  line L743 (-68.5, -37.5) -> (-82.5, -37.5)
  line L744 (-82.5, -22.5) -> (-82.5, -36.5)
  line L745 (-82.5, -36.5) -> (-68.5, -36.5)
  line L746 (-68.5, -36.5) -> (-68.5, -22.5)
  line L747 (-68.5, -22.5) -> (-82.5, -22.5)
  line L748 (-82.5, -7.5) -> (-82.5, -21.5)
  line L749 (-82.5, -21.5) -> (-68.5, -21.5)
  line L750 (-68.5, -21.5) -> (-68.5, -7.5)
  line L751 (-68.5, -7.5) -> (-82.5, -7.5)
  line L752 (-82.5, 7.5) -> (-82.5, -6.5)
  line L753 (-82.5, -6.5) -> (-68.5, -6.5)
  line L754 (-68.5, -6.5) -> (-68.5, 7.5)
  line L755 (-68.5, 7.5) -> (-82.5, 7.5)
  line L756 (-82.5, 22.5) -> (-82.5, 8.5)
  line L757 (-82.5, 8.5) -> (-68.5, 8.5)
  line L758 (-68.5, 8.5) -> (-68.5, 22.5)
  line L759 (-68.5, 22.5) -> (-82.5, 22.5)
  line L760 (-82.5, 37.5) -> (-82.5, 23.5)
  line L761 (-82.5, 23.5) -> (-68.5, 23.5)
  line L762 (-68.5, 23.5) -> (-68.5, 37.5)
  line L763 (-68.5, 37.5) -> (-82.5, 37.5)
  line L764 (-82.5, 52.5) -> (-82.5, 38.5)
  line L765 (-82.5, 38.5) -> (-68.5, 38.5)
  line L766 (-68.5, 38.5) -> (-68.5, 52.5)
  line L767 (-68.5, 52.5) -> (-82.5, 52.5)
  line L768 (-82.5, 67.5) -> (-82.5, 53.5)
  line L769 (-82.5, 53.5) -> (-68.5, 53.5)
  line L770 (-68.5, 53.5) -> (-68.5, 67.5)
  line L771 (-68.5, 67.5) -> (-82.5, 67.5)
  line L772 (-82.5, 82.5) -> (-82.5, 68.5)
  line L773 (-82.5, 68.5) -> (-68.5, 68.5)
  line L774 (-68.5, 68.5) -> (-68.5, 82.5)
  line L775 (-68.5, 82.5) -> (-82.5, 82.5)
  line L776 (-82.5, 97.5) -> (-82.5, 83.5)
  line L777 (-82.5, 83.5) -> (-68.5, 83.5)
  line L778 (-68.5, 83.5) -> (-68.5, 97.5)
  line L779 (-68.5, 97.5) -> (-82.5, 97.5)
  line L780 (-82.5, 112.5) -> (-82.5, 98.5)
  line L781 (-82.5, 98.5) -> (-68.5, 98.5)
  line L782 (-68.5, 98.5) -> (-68.5, 112.5)
  line L783 (-68.5, 112.5) -> (-82.5, 112.5)
  line L784 (-97.5, -97.5) -> (-97.5, -111.5)
  line L785 (-97.5, -111.5) -> (-83.5, -111.5)
  line L786 (-83.5, -111.5) -> (-83.5, -97.5)
  line L787 (-83.5, -97.5) -> (-97.5, -97.5)
  line L788 (-97.5, -82.5) -> (-97.5, -96.5)
  line L789 (-97.5, -96.5) -> (-83.5, -96.5)
  line L790 (-83.5, -96.5) -> (-83.5, -82.5)
  line L791 (-83.5, -82.5) -> (-97.5, -82.5)
  line L792 (-97.5, -67.5) -> (-97.5, -81.5)
  line L793 (-97.5, -81.5) -> (-83.5, -81.5)
  line L794 (-83.5, -81.5) -> (-83.5, -67.5)
  line L795 (-83.5, -67.5) -> (-97.5, -67.5)
  line L796 (-97.5, -52.5) -> (-97.5, -66.5)
  line L797 (-97.5, -66.5) -> (-83.5, -66.5)
  line L798 (-83.5, -66.5) -> (-83.5, -52.5)
  line L799 (-83.5, -52.5) -> (-97.5, -52.5)
  line L800 (-97.5, -37.5) -> (-97.5, -51.5)
  line L801 (-97.5, -51.5) -> (-83.5, -51.5)
  line L802 (-83.5, -51.5) -> (-83.5, -37.5)
  line L803 (-83.5, -37.5) -> (-97.5, -37.5)
  line L804 (-97.5, -22.5) -> (-97.5, -36.5)
  line L805 (-97.5, -36.5) -> (-83.5, -36.5)
  line L806 (-83.5, -36.5) -> (-83.5, -22.5)
  line L807 (-83.5, -22.5) -> (-97.5, -22.5)
  line L808 (-97.5, -7.5) -> (-97.5, -21.5)
  line L809 (-97.5, -21.5) -> (-83.5, -21.5)
  line L810 (-83.5, -21.5) -> (-83.5, -7.5)
  line L811 (-83.5, -7.5) -> (-97.5, -7.5)
  line L812 (-97.5, 7.5) -> (-97.5, -6.5)
  line L813 (-97.5, -6.5) -> (-83.5, -6.5)
  line L814 (-83.5, -6.5) -> (-83.5, 7.5)
  line L815 (-83.5, 7.5) -> (-97.5, 7.5)
  line L816 (-97.5, 22.5) -> (-97.5, 8.5)
  line L817 (-97.5, 8.5) -> (-83.5, 8.5)
  line L818 (-83.5, 8.5) -> (-83.5, 22.5)
  line L819 (-83.5, 22.5) -> (-97.5, 22.5)
  line L820 (-97.5, 37.5) -> (-97.5, 23.5)
  line L821 (-97.5, 23.5) -> (-83.5, 23.5)
  line L822 (-83.5, 23.5) -> (-83.5, 37.5)
  line L823 (-83.5, 37.5) -> (-97.5, 37.5)
  line L824 (-97.5, 52.5) -> (-97.5, 38.5)
  line L825 (-97.5, 38.5) -> (-83.5, 38.5)
  line L826 (-83.5, 38.5) -> (-83.5, 52.5)
  line L827 (-83.5, 52.5) -> (-97.5, 52.5)
  line L828 (-97.5, 67.5) -> (-97.5, 53.5)
  line L829 (-97.5, 53.5) -> (-83.5, 53.5)
  line L830 (-83.5, 53.5) -> (-83.5, 67.5)
  line L831 (-83.5, 67.5) -> (-97.5, 67.5)
  line L832 (-97.5, 82.5) -> (-97.5, 68.5)
  line L833 (-97.5, 68.5) -> (-83.5, 68.5)
  line L834 (-83.5, 68.5) -> (-83.5, 82.5)
  line L835 (-83.5, 82.5) -> (-97.5, 82.5)
  line L836 (-97.5, 97.5) -> (-97.5, 83.5)
  line L837 (-97.5, 83.5) -> (-83.5, 83.5)
  line L838 (-83.5, 83.5) -> (-83.5, 97.5)
  line L839 (-83.5, 97.5) -> (-97.5, 97.5)
  line L840 (-97.5, 112.5) -> (-97.5, 98.5)
  line L841 (-97.5, 98.5) -> (-83.5, 98.5)
  line L842 (-83.5, 98.5) -> (-83.5, 112.5)
  line L843 (-83.5, 112.5) -> (-97.5, 112.5)
  line L844 (-112.5, -97.5) -> (-112.5, -111.5)
  line L845 (-112.5, -111.5) -> (-98.5, -111.5)
  line L846 (-98.5, -111.5) -> (-98.5, -97.5)
  line L847 (-98.5, -97.5) -> (-112.5, -97.5)
  line L848 (-112.5, -82.5) -> (-112.5, -96.5)
  line L849 (-112.5, -96.5) -> (-98.5, -96.5)
  line L850 (-98.5, -96.5) -> (-98.5, -82.5)
  line L851 (-98.5, -82.5) -> (-112.5, -82.5)
  line L852 (-112.5, -67.5) -> (-112.5, -81.5)
  line L853 (-112.5, -81.5) -> (-98.5, -81.5)
  line L854 (-98.5, -81.5) -> (-98.5, -67.5)
  line L855 (-98.5, -67.5) -> (-112.5, -67.5)
  line L856 (-112.5, -52.5) -> (-112.5, -66.5)
  line L857 (-112.5, -66.5) -> (-98.5, -66.5)
  line L858 (-98.5, -66.5) -> (-98.5, -52.5)
  line L859 (-98.5, -52.5) -> (-112.5, -52.5)
  line L860 (-112.5, -37.5) -> (-112.5, -51.5)
  line L861 (-112.5, -51.5) -> (-98.5, -51.5)
  line L862 (-98.5, -51.5) -> (-98.5, -37.5)
  line L863 (-98.5, -37.5) -> (-112.5, -37.5)
  line L864 (-112.5, -22.5) -> (-112.5, -36.5)
  line L865 (-112.5, -36.5) -> (-98.5, -36.5)
  line L866 (-98.5, -36.5) -> (-98.5, -22.5)
  line L867 (-98.5, -22.5) -> (-112.5, -22.5)
  line L868 (-112.5, -7.5) -> (-112.5, -21.5)
  line L869 (-112.5, -21.5) -> (-98.5, -21.5)
  line L870 (-98.5, -21.5) -> (-98.5, -7.5)
  line L871 (-98.5, -7.5) -> (-112.5, -7.5)
  line L872 (-112.5, 7.5) -> (-112.5, -6.5)
  line L873 (-112.5, -6.5) -> (-98.5, -6.5)
  line L874 (-98.5, -6.5) -> (-98.5, 7.5)
  line L875 (-98.5, 7.5) -> (-112.5, 7.5)
  line L876 (-112.5, 22.5) -> (-112.5, 8.5)
  line L877 (-112.5, 8.5) -> (-98.5, 8.5)
  line L878 (-98.5, 8.5) -> (-98.5, 22.5)
  line L879 (-98.5, 22.5) -> (-112.5, 22.5)
  line L880 (-112.5, 37.5) -> (-112.5, 23.5)
  line L881 (-112.5, 23.5) -> (-98.5, 23.5)
  line L882 (-98.5, 23.5) -> (-98.5, 37.5)
  line L883 (-98.5, 37.5) -> (-112.5, 37.5)
  line L884 (-112.5, 52.5) -> (-112.5, 38.5)
  line L885 (-112.5, 38.5) -> (-98.5, 38.5)
  line L886 (-98.5, 38.5) -> (-98.5, 52.5)
  line L887 (-98.5, 52.5) -> (-112.5, 52.5)
  line L888 (-112.5, 67.5) -> (-112.5, 53.5)
  line L889 (-112.5, 53.5) -> (-98.5, 53.5)
  line L890 (-98.5, 53.5) -> (-98.5, 67.5)
  line L891 (-98.5, 67.5) -> (-112.5, 67.5)
  line L892 (-112.5, 82.5) -> (-112.5, 68.5)
  line L893 (-112.5, 68.5) -> (-98.5, 68.5)
  line L894 (-98.5, 68.5) -> (-98.5, 82.5)
  line L895 (-98.5, 82.5) -> (-112.5, 82.5)
  line L896 (-112.5, 97.5) -> (-112.5, 83.5)
  line L897 (-112.5, 83.5) -> (-98.5, 83.5)
  line L898 (-98.5, 83.5) -> (-98.5, 97.5)
  line L899 (-98.5, 97.5) -> (-112.5, 97.5)
  line L900 (-112.5, 112.5) -> (-112.5, 98.5)
  line L901 (-112.5, 98.5) -> (-98.5, 98.5)
  line L902 (-98.5, 98.5) -> (-98.5, 112.5)
  line L903 (-98.5, 112.5) -> (-112.5, 112.5)
  circle A0 centre (0, 0) radius 117.5
  circle A1 centre (0, 0) radius 122.5
  point P0 (-50.7346, -111.5)
  point P1 (81.5, -91.4549)
  point P2 (81.5, -84.6404)
  point P3 (82.5, -83.666)
  point P4 (82.5, -90.5539)
  point P5 (96.5, 75.4586)
  point P6 (90.5539, 82.5)
  point P7 (-52.5, 110.6797)
  point P8 (-52.5, 105.119)
  point P9 (-53.5, 104.6136)
  point P10 (-53.5, 110.1998)
  point P11 (-68.5, 101.5579)
  point P12 (-72.8286, 98.5)
  point P13 (-52.5, -110.6797)
  point P14 (82.668, 83.5)
  point P15 (82.5, 83.666)
  point P16 (-83.5, -82.668)
  point P17 (-83.666, -82.5)
  dimension "d24" = 15
  dimension "d27" = 15
  dimension "d30" = 5
  constraints: 1808 end point, 3 horizontal, 2 centre point, 1 vertical, 1792 other
  measures "d24" distance of L5.end L10.end
  measures "d27" distance of L5.end L66.end
  measures "d30" radial gap between concentric circles of A0 A1
extrude "Extrusion4" add sketch "Sketch5" along normal blind 10 contours A1 L1 A0 | L1 A0 L244 L245 A1 | A0 L1 | L1 A0 L545 L546 L547 L544 L606 L607 L604 L666 L667 L669 L670 L671 L668 L730 L731 L728 L790 L791 L793 L794 L795 L797 L798 L799 L796 L858 L859 L861 L862 L863 L865 L866 L867 L864 L2 L880 L881 L882 L883 L885 L886 L887 L889 L890 L828 L829 L830 L831 L833 L834 L835 L776 L777 L778 L716 L717 L718 L719 L721 L722 L660 L661 L662 L600 L601 L602 L603 L7 L363 L360 L361 L362 L300 L301 L302 L240 L241 L239 L236 L237 L238 L176 L177 L178 L116 L117 L115 L112 L113 L111 L108 L109 L110 L48 L49 L47 L44 L45 L43 L40 L41 L42 L23 L20 L21 L19 L16 L75 L72 L73 L71 L68 L130 L131 L128 L187 L184 L246 L247 L244 | A1 L605 L606 A0 L544 L545 L1 | L245 L244 A0 L246 A1 | L244 L247 L246 A0 | A1 L604 A0 L606 L605 | L246 A0 L184 A1 | A1 L2 A0 | L2 A0 L864 L865 L863 L860 A1 | A1 L666 A0 L604 | L184 A0 L187 L186 A1 | L184 L187 A0 | A0 L2 | A1 L884 L885 A0 L883 L880 L2 | L860 L863 A0 L861 A1 | A0 L604 L607 L606 | A1 L664 L667 A0 L666 | L186 L187 A0 L128 L129 A1 L127 L124 | A0 L865 L864 | L864 L867 L866 L865 A0 | A1 L887 A0 L885 L884 | L861 A0 L859 A1 | A0 L667 L666 | A1 L726 L727 L729 L730 A0 L668 L669 L667 L664 | L124 L127 A1 | A0 L130 A1 L129 L128 | L128 L131 L130 A0 | A0 L883 L882 L881 L880 | L880 L883 A0 | A1 L7 A0 | L7 A0 L603 L600 L662 L663 A1 | A1 L889 A0 L887 | L863 L862 L861 A0 | L859 A0 L858 L857 A1 | A1 L727 L726 | A0 L68 A1 L130 | A0 L7 | A1 L303 L300 A0 L362 L363 L7 | L663 L662 A0 L660 A1 | A0 L887 L886 L885 | A1 L891 L890 A0 L889 | L859 L858 A0 | L857 L858 A0 L796 L797 L795 L792 A1 L854 L855 | A0 L71 A1 L68 | L68 L71 A0 | A0 L600 L603 | L603 L602 L601 L600 A0 | A1 L302 A0 L300 L303 | L660 A0 L722 A1 | A0 L890 L889 | A1 L893 L894 L832 L833 A0 L831 L828 L890 L891 | L855 L854 A1 | A1 L728 A0 L730 L729 | A0 L73 A1 L71 | A0 L362 L361 L360 L363 | L363 L362 A0 | A1 L240 A0 L302 | L662 L661 L660 A0 | L722 A0 L721 L720 A1 | A1 L894 L893 | A0 L797 L796 | L796 L799 L798 L797 A0 | A0 L728 L731 L730 | A1 L790 A0 L728 | A0 L75 L74 A1 L73 | L73 L72 L75 A0 | A0 L302 L301 L300 | A1 L242 L241 A0 L240 | L722 L721 A0 | L720 L721 A0 L719 L716 L778 L779 A1 L781 L782 | A0 L831 L830 L829 L828 | L828 L831 A0 | L792 L795 A0 L793 A1 | A1 L791 A0 L790 | A0 L16 L17 A1 L15 L12 L74 L75 | A0 L241 L240 | A1 L180 L181 L179 L176 A0 L238 L239 L241 L242 | L782 L781 A1 | A1 L835 A0 L833 L832 | L795 L794 L793 A0 | L793 A0 L791 A1 | A0 L19 A1 L17 L16 | L16 L19 A0 | A1 L181 L180 | A0 L716 L719 | L719 L718 L717 L716 A0 | A0 L835 L834 L833 | A1 L837 L838 L776 A0 L835 | L12 L15 A1 | A0 L21 A1 L19 | A0 L238 L237 L236 L239 | L239 L238 A0 | L779 L778 A0 L776 A1 | A1 L838 L837 | A0 L23 L22 A1 L21 | L21 L20 L23 A0 | A1 L178 A0 L176 L179 | L778 L777 L776 A0 | A0 L42 L43 L45 L46 A1 L22 L23 | A0 L178 L177 L176 | A1 L116 A0 L178 | A1 L117 A0 L116 | A1 L115 A0 L117 | L46 L45 A0 L47 A1 | A1 L114 L113 A0 L115 | L47 A0 L49 A1 | L45 L44 L47 A0 | A0 L113 L112 L115 | A1 L52 L53 L51 L48 A0 L110 L111 L113 L114 | L49 A0 L48 L51 A1 | A1 L53 L52 | L49 L48 A0 | A0 L110 L109 L108 L111 | L111 L110 A0
sketch "Sketch6" plane through (0, 0, 10) normal (0, 0, 1) x (1, 0, 0)
  point P0 (0, 0)
sketch "Sketch7" plane through (0, 0, 0) normal (0, 0, -1) x (-1, 0, 0)
  line L0 (97.5, -52.5) -> (97.5, -66.5) projected
  line L1 (97.5, -66.5) -> (83.5, -66.5) projected
  line L2 (83.5, -66.5) -> (83.5, -52.5) projected
  line L3 (83.5, -52.5) -> (97.5, -52.5) projected
  line L4 (112.5, -22.5) -> (112.5, -36.5) projected
  line L5 (112.5, -36.5) -> (98.5, -36.5) projected
  line L6 (98.5, -36.5) -> (98.5, -22.5) projected
  line L7 (98.5, -22.5) -> (112.5, -22.5) projected
  line L8 (98.5, 37.5) -> (112.5, 37.5) projected
  line L9 (98.5, 23.5) -> (98.5, 37.5) projected
  line L10 (112.5, 23.5) -> (98.5, 23.5) projected
  line L11 (112.5, 37.5) -> (112.5, 23.5) projected
  line L12 (83.5, 67.5) -> (97.5, 67.5) projected
  line L13 (97.5, 67.5) -> (97.5, 53.5) projected
  line L14 (97.5, 53.5) -> (83.5, 53.5) projected
  line L15 (83.5, 53.5) -> (83.5, 67.5) projected
  line L16 (67.5, 97.5) -> (67.5, 83.5) projected
  line L17 (67.5, 83.5) -> (53.5, 83.5) projected
  line L18 (53.5, 83.5) -> (53.5, 97.5) projected
  line L19 (53.5, 97.5) -> (67.5, 97.5) projected
  line L20 (23.5, 112.5) -> (37.5, 112.5) projected
  line L21 (23.5, 98.5) -> (23.5, 112.5) projected
  line L22 (37.5, 98.5) -> (23.5, 98.5) projected
  line L23 (37.5, 112.5) -> (37.5, 98.5) projected
  line L24 (-36.5, 112.5) -> (-22.5, 112.5) projected
  line L25 (-22.5, 112.5) -> (-22.5, 98.5) projected
  line L26 (-22.5, 98.5) -> (-36.5, 98.5) projected
  line L27 (-36.5, 98.5) -> (-36.5, 112.5) projected
  line L28 (-66.5, 97.5) -> (-52.5, 97.5) projected
  line L29 (-52.5, 97.5) -> (-52.5, 83.5) projected
  line L30 (-52.5, 83.5) -> (-66.5, 83.5) projected
  line L31 (-66.5, 83.5) -> (-66.5, 97.5) projected
  line L32 (-96.5, 67.5) -> (-82.5, 67.5) projected
  line L33 (-82.5, 67.5) -> (-82.5, 53.5) projected
  line L34 (-82.5, 53.5) -> (-96.5, 53.5) projected
  line L35 (-96.5, 53.5) -> (-96.5, 67.5) projected
  point P0 (0, 0)
extrude "Extrusion5" cut sketch "Sketch7" against normal blind 47.25
body "Solid4"
